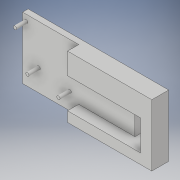
# Autodesk Inventor part: Case
Saved by Autodesk Inventor 2017 (Build 210142000, 142)
## iProperties
Created: 2016-11-30
Part Number: Case
Material: Generic
Document SubType Name: Modeling
Designer: SDL
Density: 1 g/cm^3
Appearance: Default
Author: SDL
Autodesk Inventor part; units mm, degrees
ref_plane "YZ Plane" through (0, 0, 0) normal (1, 0, 0) x (0, 1, 0)
ref_plane "XZ Plane" through (0, 0, 0) normal (0, 1, 0) x (-1, 0, 0)
ref_plane "XY Plane" through (0, 0, 0) normal (0, 0, 1) x (1, 0, 0)
sketch "Sketch3" plane through (0, 0, 0) normal (0, 0, 1) x (1, 0, 0)
  line L0 (0, 0) -> (125, 0)
  line L1 (125, 0) -> (125, 55)
  line L2 (125, 55) -> (0, 55)
  line L3 (0, 55) -> (0, 0)
  dimension "d0" = 125
  dimension "d1" = 55
  constraints: 8 end point, 2 parallel, 1 horizontal, 1 perpendicular
  measures "d0" distance of L2.end L1.end
  measures "d1" distance of L1.end L0.end
extrude "Extrusion1" add sketch "Sketch3" along normal blind 5
sketch "Sketch6" plane through (0, 0, 5) normal (0, 0, 1) x (1, 0, 0)
  line L0 (0, 55) -> (0, 0) projected
  line L1 (0, 27.5) -> (125, 27.5)
  line L2 (125, 0) -> (125, 55) projected
  line L3 (0, 27.5) -> (0, 52.5)
  line L4 (0, 27.5) -> (0, 2.5)
  line L5 (0, 2.5) -> (50, 2.5)
  line L6 (50, 2.5) -> (50, 52.5)
  line L7 (50, 52.5) -> (0, 52.5)
  line L8 (0, 52.5) -> (0, 49.5)
  line L9 (0, 49.5) -> (3.2, 49.5)
  line L10 (0, 2.5) -> (0, 19.2)
  line L11 (0, 2.5) -> (16.7, 2.5) construction
  line L12 (0, 19.2) -> (14.3, 19.2)
  line L13 (50, 2.5) -> (41.9, 2.5)
  line L14 (41.9, 2.5) -> (41.9, 15)
  circle A0 centre (3.2, 49.5) radius 1.45
  circle A1 centre (14.3, 19.2) radius 1.45
  circle A2 centre (41.9, 15) radius 1.45
  dimension "d4" = 25
  dimension "d5" = 25
  dimension "d6" = 50
  dimension "d7" = 50
  dimension "d8" = 3
  dimension "d9" = 3.2
  dimension "d10" = 16.7
  dimension "d11" = 90
  dimension "d12" = 14.3
  dimension "d13" = 8.1
  dimension "d14" = 12.5
  dimension "d15" = 2.9
  dimension "d16" = 2.9
  dimension "d17" = 2.9
  constraints: 26 end point, 6 perpendicular, 4 point on line, 3 centre point, 3 coincident, 2 midpoint, 1 horizontal, 1 vertical
  measures "d4" distance of L1.start L3.end
  measures "d5" distance of L1.start L4.end
  measures "d6" distance of L4.end L5.end
  measures "d7" distance of L5.end L6.end
  measures "d8" distance of L3.end L8.end
  measures "d9" distance of L8.end L9.end
  measures "d10" distance of L4.end L10.end
  measures "d11" angle of L11 L10
  measures "d12" distance of L10.end L12.end
  measures "d13" distance of L5.end L13.end
  measures "d14" distance of L13.end L14.end
  measures "d15" diameter of A0
  measures "d16" diameter of A1
  measures "d17" diameter of A2
extrude "Extrusion2" add sketch "Sketch6" along normal blind 10 contours A0 | A1 | A2
sketch "Sketch7" plane through (0, 0, 5) normal (0, 0, 1) x (1, 0, 0)
  line L0 (125, 0) -> (125, 55) projected
  line L1 (0, 0) -> (125, 0) projected
  line L2 (125, 55) -> (50, 55)
  line L3 (50, 55) -> (50, 0)
  line L4 (50, 0) -> (125, 0)
  line L5 (125, 0) -> (125, 55)
  dimension "d20" = 75
  constraints: 8 end point, 2 parallel, 1 horizontal, 1 perpendicular, 1 point on line
  measures "d20" distance of L4.end L3.end
extrude "Extrusion3" add sketch "Sketch7" along normal blind 10
sketch "Sketch8" plane through (0, 0, 15) normal (0, 0, 1) x (1, 0, 0)
  line L0 (50, 55) -> (50, 0) projected
  line L1 (50, 0) -> (50, 9)
  line L2 (50, 9) -> (115, 9)
  line L3 (115, 9) -> (115, 36)
  line L4 (115, 36) -> (50, 36)
  line L5 (50, 36) -> (50, 9)
  point P0 (0, 0)
  dimension "d23" = 9
  dimension "d24" = 65
  dimension "d25" = 27
  constraints: 10 end point, 2 parallel, 1 horizontal, 1 perpendicular, 1 point on line
  measures "d23" distance of L0.end L1.end
  measures "d24" distance of L4.end L3.end
  measures "d25" distance of L3.end L2.end
extrude "Extrusion4" cut sketch "Sketch8" against normal blind 10
sketch "Sketch9" plane through (0, 0, 15) normal (0, 0, 1) x (1, 0, 0)
  line L0 (50, 36) -> (115, 36) projected
  line L1 (115, 9) -> (50, 9) projected
  line L2 (115, 36) -> (100, 36)
  line L3 (100, 36) -> (100, 9)
  line L4 (100, 9) -> (115, 9)
  line L5 (115, 9) -> (115, 36)
  point P0 (0, 0)
  dimension "d28" = 15
  constraints: 8 end point, 2 parallel, 1 horizontal, 1 perpendicular, 1 point on line
  measures "d28" distance of L4.end L3.end
extrude "Extrusion5" cut sketch "Sketch9" against normal blind 20
body "Solid1"
